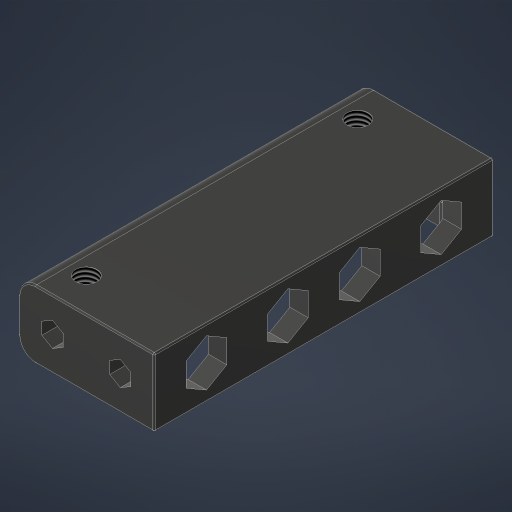
# Autodesk Inventor part: EL2-017
Saved by Autodesk Inventor 2023.4 (Build 274418000, 418)
## iProperties
Created: 2025-01-21
Part Number: EL2-017
Material: Thermoplastic Resin
Document SubType Name: Modeling
Designer: slick
Density: 1.28 g/cm^3
Appearance: Smooth - Black
Author: slick
Autodesk Inventor part; units mm, degrees
ref_plane "YZ Plane" through (0, 0, 0) normal (1, 0, 0) x (0, 1, 0)
ref_plane "XZ Plane" through (0, 0, 0) normal (0, 1, 0) x (-1, 0, 0)
ref_plane "XY Plane" through (0, 0, 0) normal (0, 0, 1) x (1, 0, 0)
sketch "Sketch1" plane through (0, 0, 0) normal (0, 0, 1) x (1, 0, 0)
  line L0 (-12.7, 6.35) -> (12.7, 6.35)
  line L1 (12.7, 6.35) -> (12.7, -6.35)
  line L2 (12.7, -6.35) -> (-12.7, -6.35)
  line L3 (-12.7, -6.35) -> (-12.7, 6.35)
  line L4 (-12.7, 6.35) -> (12.7, -6.35) construction
  line L5 (12.7, 6.35) -> (-12.7, -6.35) construction
  point P0 (0, 0)
  dimension "d0" = 25.4
  dimension "d1" = 12.7
  constraints: 12 end point, 2 midpoint, 2 parallel, 1 horizontal, 1 perpendicular
  measures "d0" distance of L1.end L2.end
  measures "d1" distance of L0.end L1.end
extrude "Extrusion1" add sketch "Sketch1" along normal mid plane 63.5
sketch "Sketch2" plane through (-12.7, 6.35, 31.75) normal (0, 1, 0) x (1, 0, 0)
  line L0 (6.35, 57.15) -> (6.35, 6.35) construction
  line L1 (0, 63.5) -> (0, 0) projected
  point P0 (12.7, 31.75)
  point P1 (6.35, 31.75)
  dimension "d4" = 50.8
  dimension "d5" = 6.35
  constraints: 2 end point, 1 horizontal alignment, 1 midpoint, 1 vertical, 1 vertical alignment
  measures "d4" distance of L0.start L0.end
  measures "d5" distance between parallel lines of L1 L0
hole "Hole1" at (-6.35, 6.35, 25.4) at (-6.35, 6.35, -25.4) direction (0, -1, 0) diameter 3.9624 end through all thread size "10-32 UNF" class "2B" standard "ANSI Unified Screw Threads"
fillet "Fillet1" radius 3.175 2 edges at (-12.7, 6.35, 0) (-12.7, -6.35, 0)
fillet "Fillet2" radius 0.254 14 edges at (-11.7701, 5.4201, 31.75) (-12.7, 0, 31.75) (-11.7701, -5.4201, 31.75) (1.5875, -6.35, 31.75) (1.5875, 6.35, 31.75) (12.7, 6.35, 0) (12.7, -6.35, 0) (12.7, 0, -31.75) (12.7, 0, 31.75) (-11.7701, 5.4201, -31.75) (-12.7, 0, -31.75) (-11.7701, -5.4201, -31.75) (1.5875, -6.35, -31.75) (1.5875, 6.35, -31.75)
sketch "Sketch3" plane through (-9.525, -6.35, 31.496) normal (0, -1, 0) x (1, 0, 0)
  line L0 (21.971, -62.992) -> (21.971, 0) projected
  line L1 (0, 0) -> (21.971, 0) projected
  line L2 (0, 0) -> (0, -62.992) projected
  line L3 (21.971, -62.992) -> (0, -62.992) projected
  circle A0 centre (3.175, -6.096) radius 1.9812 projected
  circle A1 centre (3.175, -56.896) radius 1.9812 projected
  line L4 (18.796, -3.175) -> (18.796, -59.817)
  line L5 (18.796, -59.817) -> (3.175, -59.817) construction
  line L6 (3.175, -59.817) -> (3.175, -3.175) construction
  line L7 (3.175, -3.175) -> (18.796, -3.175) construction
  circle A2 centre (3.175, -6.096) radius 5.1562 construction
  circle A3 centre (3.175, -56.896) radius 5.1562 construction
  line L8 (18.796, -3.175) -> (7.424, -3.175)
  line L9 (7.424, -59.817) -> (18.796, -59.817)
  arc A4 (0, -10.1587) -> (7.424, -3.175) centre (3.175, -6.096) ccw
  circle A5 centre (3.175, -56.896) radius 1.9812 projected
  arc A6 (7.424, -59.817) -> (0, -52.8333) centre (3.175, -56.896) ccw
  line L10 (21.971, -62.992) -> (21.971, 0) construction
  line L11 (0, 0) -> (21.971, 0) construction
  line L12 (0, 0) -> (0, -62.992) construction
  line L13 (21.971, -62.992) -> (0, -62.992) construction
  circle A7 centre (3.175, -6.096) radius 1.9812 construction
  circle A8 centre (3.175, -56.896) radius 1.9812 construction
  line L14 (0, 0) -> (0, -62.992) projected
  line L15 (0, -52.8333) -> (0, -10.1587)
  point P0 (9.525, -31.496)
  point P1 (0, -52.8333)
  dimension "d15" = 3.175
  dimension "d16" = 3.175
  dimension "d17" = 3.175
  constraints: 14 end point, 8 point on circle, 4 centre point, 4 point on line, 2 coincident, 3 other
  measures "d15" distance between parallel lines of L0 L4
  measures "d16" radial gap between concentric circles of A0 A2
  measures "d17" radial gap between concentric circles of A1 A3
extrude "Extrusion2" cut sketch "Sketch3" against normal blind 9.525 contours L2 A4 L8 L4 L9 A6
fillet "Fillet3" radius 3.302 6 edges at (-2.101, -1.5875, 28.321) (9.271, -1.5875, 28.321) (9.271, -1.5875, -28.321) (-2.101, -1.5875, -28.321) (-9.525, -1.5875, -21.3373) (-9.525, -1.5875, 21.3373)
sketch "Sketch4" plane through (12.7, -6.096, 31.496) normal (1, 0, 0) x (0, 0, -1)
  line L0 (9.525, 10.4954) -> (13.335, 8.2957)
  line L1 (13.335, 8.2957) -> (13.335, 3.8963)
  line L2 (13.335, 3.8963) -> (9.525, 1.6966)
  line L3 (9.525, 1.6966) -> (5.715, 3.8963)
  line L4 (5.715, 3.8963) -> (5.715, 8.2957)
  line L5 (5.715, 8.2957) -> (9.525, 10.4954)
  line L6 (0, 0) -> (0, 12.192) construction
  line L7 (0, 12.192) -> (62.992, 12.192) construction
  line L8 (24.765, 10.4954) -> (28.575, 8.2957)
  line L9 (28.575, 8.2957) -> (28.575, 3.8963)
  line L10 (28.575, 3.8963) -> (24.765, 1.6966)
  line L11 (24.765, 1.6966) -> (20.955, 3.8963)
  line L12 (20.955, 3.8963) -> (20.955, 8.2957)
  line L13 (20.955, 8.2957) -> (24.765, 10.4954)
  line L14 (31.496, 12.192) -> (31.496, -0.254) construction
  line L15 (0, -0.254) -> (62.992, -0.254) construction
  line L16 (53.467, 10.4954) -> (49.657, 8.2957)
  line L17 (49.657, 8.2957) -> (49.657, 3.8963)
  line L18 (49.657, 3.8963) -> (53.467, 1.6966)
  line L19 (53.467, 1.6966) -> (57.277, 3.8963)
  line L20 (57.277, 3.8963) -> (57.277, 8.2957)
  line L21 (57.277, 8.2957) -> (53.467, 10.4954)
  line L22 (38.227, 10.4954) -> (34.417, 8.2957)
  line L23 (34.417, 8.2957) -> (34.417, 3.8963)
  line L24 (34.417, 3.8963) -> (38.227, 1.6966)
  line L25 (38.227, 1.6966) -> (42.037, 3.8963)
  line L26 (42.037, 3.8963) -> (42.037, 8.2957)
  line L27 (42.037, 8.2957) -> (38.227, 10.4954)
  point P0 (31.496, 6.096)
  point P1 (9.525, 6.096)
  point P2 (13.335, 6.096)
  point P3 (5.715, 6.096)
  point P4 (24.765, 6.096)
  point P5 (28.575, 6.096)
  point P6 (20.955, 6.096)
  point P7 (53.467, 6.096)
  point P8 (49.657, 6.096)
  point P9 (57.277, 6.096)
  point P10 (38.227, 6.096)
  point P11 (34.417, 6.096)
  point P12 (42.037, 6.096)
  dimension "d21" = 7.62
  dimension "d22" = 9.525
  dimension "d25" = 15.24
  constraints: 50 end point, 18 symmetric about line, 4 midpoint, 1 horizontal, 1 horizontal alignment, 1 vertical, 28 other
  measures "d21" distance of point (13.335, 6.096) point (5.715, 6.096)
  measures "d22" distance from line of L6 point (9.525, 6.096)
  measures "d25" distance of point (9.525, 6.096) point (24.765, 6.096)
extrude "Extrusion3" cut sketch "Sketch4" against normal through all
sketch "Sketch5" plane through (0, 0, 31.75) normal (0, 0, 1) x (1, 0, 0)
  line L0 (-4.3688, -6.35) -> (-4.3688, 6.35) construction
  line L1 (-4.3688, 1.1438) -> (-4.3688, -1.1438)
  line L2 (-4.3688, -1.1438) -> (-6.35, -2.2877)
  line L3 (-6.35, -2.2877) -> (-8.3312, -1.1438)
  line L4 (-8.3312, -1.1438) -> (-8.3312, 1.1438)
  line L5 (-8.3312, 1.1438) -> (-6.35, 2.2877)
  line L6 (-6.35, 2.2877) -> (-4.3688, 1.1438)
  line L7 (0, 6.096) -> (0, -7.4763) construction
  line L8 (-9.525, 6.096) -> (12.446, 6.096) construction
  line L9 (4.3688, 1.1438) -> (4.3688, -1.1438)
  line L10 (4.3688, -1.1438) -> (6.35, -2.2877)
  line L11 (6.35, -2.2877) -> (8.3312, -1.1438)
  line L12 (8.3312, -1.1438) -> (8.3312, 1.1438)
  line L13 (8.3312, 1.1438) -> (6.35, 2.2877)
  line L14 (6.35, 2.2877) -> (4.3688, 1.1438)
  point P0 (0, 0)
  point P1 (-6.35, 0)
  point P2 (0, -0.6901)
  point P3 (6.35, 0)
  dimension "d32" = 6.35
  constraints: 26 end point, 7 symmetric about line, 2 point on line, 2 vertical, 1 horizontal alignment, 1 midpoint, 1 vertical alignment, 13 other
  measures "d32" distance from line of L7 point (-6.35, 0)
extrude "Extrusion4" cut sketch "Sketch5" against normal through all
body "Solid1"
